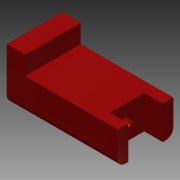
# Autodesk Inventor part: Carcasa (parte 2)
Saved by Autodesk Inventor 2014 (Build 180170000, 170)
## iProperties
Created: 2017-02-07
Part Number: Carcasa (parte 2)
Material: Generic
Document SubType Name: Modeling
Designer: Rubén
Density: 1 g/cm^3
Appearance: Red
Author: Rubén
Autodesk Inventor part; units mm, degrees
ref_plane "YZ Plane" through (0, 0, 0) normal (1, 0, 0) x (0, 1, 0)
ref_plane "XZ Plane" through (0, 0, 0) normal (0, 1, 0) x (-1, 0, 0)
ref_plane "XY Plane" through (0, 0, 0) normal (0, 0, 1) x (1, 0, 0)
sketch "Sketch1" plane through (0, 0, 0) normal (0, 1, 0) x (-1, 0, 0)
  line L0 (0, 0) -> (0, 4.65)
  line L1 (0, 4.65) -> (-5, 4.65)
  line L2 (-5, 4.65) -> (-5, 7.5)
  line L3 (-5, 7.5) -> (25, 7.5)
  line L4 (25, 7.5) -> (25, 0)
  line L5 (25, 0) -> (0, 0) construction
  line L6 (0, 0) -> (0, -4.65)
  line L7 (0, -4.65) -> (-5, -4.65)
  line L8 (-5, -4.65) -> (-5, -7.5)
  line L9 (-5, -7.5) -> (25, -7.5)
  line L10 (25, -7.5) -> (25, 0)
  dimension "d7" = 9.3
  dimension "d8" = 15
  dimension "d9" = 5
  dimension "d10" = 25
  constraints: 22 end point, 4 parallel, 4 symmetric about line, 1 perpendicular, 1 vertical
  measures "d7" distance between parallel lines of L7 L1
  measures "d8" distance between parallel lines of L9 L3
  measures "d9" distance of L0.end L1.end
  measures "d10" distance of L4.end L0.start
extrude "Extrusion1" add sketch "Sketch1" along normal blind 9
sketch "Sketch2" plane through (0, 9, 0) normal (0, 1, 0) x (1, 0, 0)
  line L0 (5, 7.5) -> (-25, 7.5) projected
  line L1 (-25, 7.5) -> (-25, -7.5) projected
  line L2 (-25, -7.5) -> (5, -7.5) projected
  line L3 (-20, 7.5) -> (-20, -7.5)
  point P0 (0, 0)
  dimension "d11" = 5
  constraints: 2 end point, 2 point on line, 1 perpendicular
  measures "d11" distance between parallel lines of L1 L3
extrude "Extrusion2" add sketch "Sketch2" along normal blind 5
sketch "Sketch3" plane through (0, 0, 4.65) normal (1, 0, 0) x (0, 0, -1)
  line L0 (9.3, 0) -> (9.3, 9) projected
  line L1 (0, 9) -> (9.3, 9) projected
  line L2 (0, 0) -> (0, 9) projected
  line L3 (0, 4.5) -> (9.3, 4.5) construction
  line L4 (4.65, 9) -> (4.65, 0) construction
  circle A0 centre (4.65, 4.5) radius 1.5
  dimension "d4" = 3
  constraints: 4 end point, 4 midpoint, 1 centre point, 1 perpendicular
  measures "d4" diameter of A0
extrude "Extrusion3" cut sketch "Sketch3" against normal blind 15
fillet "Fillet1" radius 2 2 edges at (-10, 0, -7.5) (-10, 0, 7.5)
body "Solid1"
